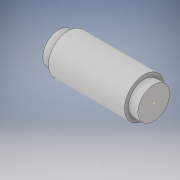
# Autodesk Inventor part: roller pin
Saved by Autodesk Inventor 2019 (Build 230136000, 136)
## iProperties
Created: 2020-02-15
Part Number: roller pin
Material: Generic
Document SubType Name: Modeling
Designer: Admin
Density: 1 g/cm^3
Appearance: Default
Author: Admin
Autodesk Inventor part; units mm, degrees
ref_plane "YZ Plane" through (0, 0, 0) normal (1, 0, 0) x (0, 1, 0)
ref_plane "XZ Plane" through (0, 0, 0) normal (0, 1, 0) x (-1, 0, 0)
ref_plane "XY Plane" through (0, 0, 0) normal (0, 0, 1) x (1, 0, 0)
sketch "Sketch1" plane through (0, 0, 0) normal (0, 0, 1) x (1, 0, 0)
  line L0 (0, 0) -> (0, 10)
  line L1 (0, 10) -> (6, 10)
  line L2 (6, 10) -> (6, 12.5)
  line L3 (6, 12.5) -> (54, 12.5)
  line L4 (54, 12.5) -> (54, 10)
  line L5 (54, 10) -> (60, 10)
  line L6 (60, 10) -> (60, 0)
  line L7 (60, 0) -> (0, 0)
  dimension "d0" = 10
  dimension "d1" = 6
  dimension "d2" = 2.5
  dimension "d3" = 48
  dimension "d4" = 2.5
  dimension "d5" = 6
  dimension "d6" = 10
  constraints: 16 end point, 4 perpendicular, 2 point on line, 1 vertical
  measures "d0" distance of L0.start L0.end
  measures "d1" distance of L0.end L1.end
  measures "d2" distance of L1.end L2.end
  measures "d3" distance of L2.end L3.end
  measures "d4" distance of L3.end L4.end
  measures "d5" distance of L4.end L5.end
  measures "d6" distance of L5.end L6.end
revolve "Revolution1" add sketch "Sketch1" angle 360 about axis through (60, 0, 0) along (-1, 0, 0)
sketch "Sketch2" plane through (60, 0, 0) normal (1, 0, 0) x (0, 0, -1)
  point P0 (0, 0)
  point P1 (-32.9803, -18.1231)
body "Solid1"
